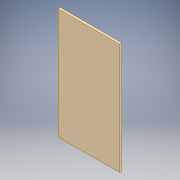
# Autodesk Inventor part: InsulatorCeiling
Saved by Autodesk Inventor 2017 (Build 210142000, 142)
## iProperties
Created: 2016-12-13
Part Number: InsulatorCeiling
Material: Polyethylene, Low Density
Document SubType Name: Modeling
Designer: umr
Density: 0.894 g/cm^3
Appearance: Smooth - Off-White
Author: umr
Autodesk Inventor part; units mm, degrees
ref_plane "YZ Plane" through (0, 0, 0) normal (1, 0, 0) x (0, 1, 0)
ref_plane "XZ Plane" through (0, 0, 0) normal (0, 1, 0) x (-1, 0, 0)
ref_plane "XY Plane" through (0, 0, 0) normal (0, 0, 1) x (1, 0, 0)
sketch "Sketch1" plane through (0, 0, 0) normal (0, 1, 0) x (-1, 0, 0)
  line L0 (0, 0) -> (1500, 0)
  line L1 (1500, 0) -> (1500, -2710)
  line L2 (1500, -2710) -> (0, -2710)
  line L3 (0, -2710) -> (0, 0)
  dimension "d0" = 1500
  dimension "d1" = 2710
  constraints: 8 end point, 2 parallel, 1 horizontal, 1 perpendicular
  measures "d0" distance of L1.end L2.end
  measures "d1" distance of L0.end L1.end
extrude "Extrusion1" add sketch "Sketch1" along normal blind 50
body "Solid1"
